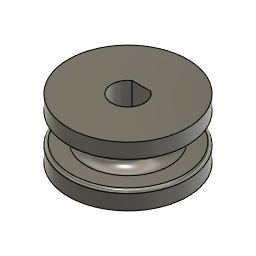
Winding Gear v4 (Autodesk Fusion 360 design; units mm, degrees)
Autodesk Fusion 360 part; units mm, degrees
sketch "Sketch1" plane through (0, 0, 0) normal (0, 1, 0) x (1, 0, 0)
  line L0 (1.5, 2) -> (-1.5, 2)
  arc A0 (-1.5, 2) -> (1.5, 2) centre (0, 0) ccw
  arc A1 (-1.5811, 2.25) -> (1.5811, 2.25) centre (0, 0) ccw
  line L1 (1.5811, 2.25) -> (-1.5811, 2.25)
  circle A2 centre (0, 0) radius 10
  dimension "d1" = 0.25
  constraint concentric A0 A2
extrude "Extrude1" add sketch "Sketch1" along normal blind 10 contours A2
ref_plane "WorkPlane1" through (0, 3, 0) normal (0, -1, 0) x (-1, 0, 0)
sketch "Sketch2" plane through (0, 3, 0) normal (0, -1, 0) x (1, 0, 0)
  line L0 (-1.5811, -2.25) -> (1.5811, -2.25)
  arc A0 (1.5811, -2.25) -> (-1.5811, -2.25) centre (0, 0) ccw
  circle A1 centre (0, 0) radius 10
  circle A2 centre (0, 0) radius 5
  constraint concentric A0 A2
extrude "Extrude2" cut sketch "Sketch2" against normal blind 4 contours A1
sketch "Sketch3" plane through (0, 3, 0) normal (0, 1, 0) x (-1, 0, 0)
  circle A0 centre (0, 0) radius 5
  circle A1 centre (0, 0) radius 10
  circle A2 centre (0, 0) radius 5
  circle A3 centre (0, 0) radius 5
  circle A4 centre (7, 0) radius 1
extrude "Extrude3" add sketch "Sketch3" along normal blind 4 contours A4
fillet "Fillet3" radius 2 2 edges at (-4.6616, 7, -1.8081) (-4.6616, 3, 1.8081)
fillet "Fillet4" radius 0.5 2 edges at (-9.3233, 3, -3.6162) (-9.3233, 7, 3.6162)
